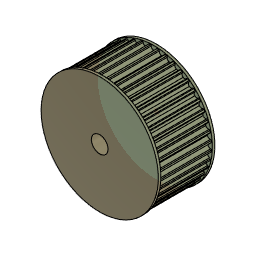
roue1 v6 (Autodesk Fusion 360 design; units mm, degrees)
Autodesk Fusion 360 part; units mm, degrees
sketch "Esquisse1" plane through (0, 0, 0) normal (0, 1, 0) x (1, 0, 0)
  circle A0 centre (0, 0) radius 35.015
  dimension "d1" = 70.03
  constraint coincident A0.centre origin
  measures "d1" diameter of A0
extrude "Extrusion1" add sketch "Esquisse1" along normal blind 1.5
sketch "Esquisse2" plane through (0, 0, 0) normal (0, 1, 0) x (1, 0, 0)
  arc A0 (-1.5243, 33.9566) -> (0, 32.385) centre (0, 33.91) ccw
  arc A1 (-29.4542, -13.4626) -> (-31.5172, -12.7295) centre (-30.8411, -14.0965) ccw
  arc A2 (-27.742, -19.6406) -> (-27.244, -17.5087) centre (-28.5269, -18.3331) ccw
  line L0 (-7.8107, 33.5477) -> (-6.8421, 33.7586)
  arc A3 (-0.0103, 32.385) -> (1.5135, 33.9571) centre (-0.0108, 33.91) ccw
  line L1 (0, 0) -> (37.4833, 0) construction
  arc A4 (-15.4926, 30.2548) -> (-16.0758, 30.4635) centre (-15.8798, 30.0921) ccw
  arc A5 (-33.9566, -1.5243) -> (-32.385, 0) centre (-33.91, 0) ccw
  line L2 (-2.9569, 34.3179) -> (-1.9681, 34.3887)
  arc A6 (-33.5477, -7.8107) -> (-33.008, -8.1146) centre (-33.1387, -7.7155) ccw
  arc A7 (33.7608, -6.8314) -> (33.396, -6.3307) centre (33.3491, -6.7481) ccw
  arc A8 (-6.3413, 33.394) -> (-6.8421, 33.7586) centre (-6.7587, 33.347) ccw
  arc A9 (-29.9883, -16.9458) -> (-29.3848, -17.0853) centre (-29.6226, -16.7392) ccw
  arc A10 (33.8279, -3.3238) -> (32.0554, -4.6089) centre (33.5648, -4.8259) ccw
  arc A11 (-13.4626, 29.4542) -> (-12.7295, 31.5172) centre (-14.0965, 30.8411) ccw
  line L3 (-33.5477, -7.8107) -> (-33.7586, -6.8421)
  arc A12 (-2.9569, 34.3179) -> (-3.3345, 33.8268) centre (-2.9208, 33.8994) ccw
  arc A13 (-32.1517, -11.0292) -> (-32.4413, -11.5768) centre (-32.0457, -11.4356) ccw
  arc A14 (-17.5173, 27.2384) -> (-17.0853, 29.3848) centre (-18.3422, 28.5211) ccw
  line L4 (-29.9883, -16.9458) -> (-30.4635, -16.0758)
  circle A15 centre (0, -33.91) radius 1.525 construction
  arc A16 (-32.385, -0.0103) -> (-33.9571, 1.5135) centre (-33.91, -0.0108) ccw
  arc A17 (33.9566, 1.5243) -> (32.385, 0) centre (33.91, 0) ccw
  arc A18 (0.0103, -32.385) -> (-1.5135, -33.9571) centre (0.0108, -33.91) ccw
  circle A19 centre (0, 0) radius 34.445 construction
  arc A20 (-30.2548, -15.4926) -> (-29.4584, -13.4532) centre (-30.8456, -14.0867) ccw
  arc A21 (3.3238, 33.8279) -> (2.946, 34.3188) centre (2.91, 33.9003) ccw
  arc A22 (9.1338, -31.0703) -> (8.1146, -33.008) centre (9.5639, -32.5334) ccw
  arc A23 (-8.1041, -33.0105) -> (-9.1239, -31.0732) centre (-9.5536, -32.5364) ccw
  arc A24 (6.3413, -33.394) -> (4.6089, -32.0554) centre (4.8259, -33.5648) ccw
  arc A25 (-24.6645, -23.3888) -> (-24.7004, -24.0072) centre (-24.3993, -23.7145) ccw
  arc A26 (31.5212, -12.7195) -> (32.0987, -12.4954) centre (31.7073, -12.343) ccw
  line L5 (34.3894, -1.9572) -> (34.3188, -2.946)
  circle A27 centre (4.8365, -33.5633) radius 1.525 construction
  arc A28 (-1.9572, -34.3894) -> (-1.5135, -33.9571) centre (-1.9333, -33.97) ccw
  arc A29 (33.8279, -3.3238) -> (34.3188, -2.946) centre (33.9003, -2.91) ccw
  arc A30 (32.4449, -11.5665) -> (32.1552, -11.019) centre (32.0493, -11.4255) ccw
  line L6 (-6.8314, -33.7608) -> (-7.8001, -33.5502)
  line L7 (-23.9994, -24.7081) -> (-24.7004, -24.0072)
  arc A31 (13.4439, 29.4627) -> (15.483, 30.2597) centre (14.0769, 30.8501) ccw
  arc A32 (15.4926, -30.2548) -> (13.4532, -29.4584) centre (14.0867, -30.8456) ccw
  line L8 (16.9458, -29.9883) -> (16.0758, -30.4635)
  arc A33 (11.5665, 32.4449) -> (11.019, 32.1552) centre (11.4255, 32.0493) ccw
  line L9 (30.4686, -16.0662) -> (29.9937, -16.9363)
  arc A34 (-17.5, -27.2496) -> (-19.6318, -27.7482) centre (-18.3241, -28.5327) ccw
  arc A35 (-26.6609, 21.0849) -> (-27.2781, 21.0324) centre (-26.9455, 20.776) ccw
  arc A36 (-27.872, 20.2388) -> (-27.7482, 19.6318) centre (-27.5322, 19.992) ccw
  arc A37 (-26.6609, 21.0849) -> (-24.4749, 21.2077) centre (-25.6275, 22.2063) ccw
  circle A38 centre (0, 0) radius 32.385 construction
  arc A39 (26.6609, -21.0849) -> (24.4749, -21.2077) centre (25.6275, -22.2063) ccw
  line L10 (27.872, -20.2388) -> (27.2781, -21.0324)
  arc A40 (26.6609, -21.0849) -> (27.2781, -21.0324) centre (26.9455, -20.776) ccw
  line L11 (0, 0) -> (5.3462, -37.1001) construction
  arc A41 (24.4817, -21.1999) -> (24.6719, -23.381) centre (25.6345, -22.1982) ccw
  arc A42 (23.3888, -24.6645) -> (21.2077, -24.4749) centre (22.2063, -25.6275) ccw
  arc A43 (-24.4817, 21.1999) -> (-24.6719, 23.381) centre (-25.6345, 22.1982) ccw
  arc A44 (19.6406, -27.742) -> (17.5087, -27.244) centre (18.3331, -28.5269) ccw
  arc A45 (19.6406, -27.742) -> (20.2476, -27.8656) centre (20.0007, -27.5258) ccw
  arc A46 (23.3888, -24.6645) -> (24.0072, -24.7004) centre (23.7145, -24.3993) ccw
  arc A47 (21.2154, -24.4682) -> (21.0933, -26.6542) centre (22.2145, -25.6204) ccw
  line L12 (0, 0) -> (0, -40) construction
  line L13 (21.0411, -27.2714) -> (20.2476, -27.8656)
  arc A48 (24.7081, -23.9994) -> (24.6719, -23.381) centre (24.4068, -23.7067) ccw
  line L14 (-27.872, 20.2388) -> (-27.2781, 21.0324)
  arc A49 (21.0411, -27.2714) -> (21.0933, -26.6542) centre (20.7845, -26.9389) ccw
  line L15 (24.7081, -23.9994) -> (24.0072, -24.7004)
  line L16 (-33.7608, 6.8314) -> (-33.5502, 7.8001)
  arc A50 (-17.076, -29.3902) -> (-16.9363, -29.9937) centre (-16.7298, -29.6279) ccw
  line L17 (-16.0662, -30.4686) -> (-16.9363, -29.9937)
  arc A51 (-3.3238, -33.8279) -> (-4.6089, -32.0554) centre (-4.8259, -33.5648) ccw
  arc A52 (16.0662, 30.4686) -> (15.483, 30.2597) centre (15.8703, 30.0971) ccw
  arc A53 (9.114, 31.0761) -> (11.019, 32.1552) centre (9.5432, 32.5394) ccw
  arc A54 (-21.1999, -24.4817) -> (-23.381, -24.6719) centre (-22.1982, -25.6345) ccw
  arc A55 (29.3902, -17.076) -> (27.244, -17.5087) centre (28.5269, -18.3331) ccw
  arc A56 (12.7195, 31.5212) -> (13.4532, 29.4584) centre (14.0867, 30.8456) ccw
  arc A57 (-21.0411, 27.2714) -> (-21.0933, 26.6542) centre (-20.7845, 26.9389) ccw
  line L18 (12.5055, -32.0947) -> (11.5768, -32.4413)
  arc A58 (-33.0105, 8.1041) -> (-33.5502, 7.8001) centre (-33.1411, 7.7049) ccw
  arc A59 (-6.8314, -33.7608) -> (-6.3307, -33.396) centre (-6.7481, -33.3491) ccw
  arc A60 (-19.6406, 27.742) -> (-17.5087, 27.244) centre (-18.3331, 28.5269) ccw
  arc A61 (-31.5212, 12.7195) -> (-29.4584, 13.4532) centre (-30.8456, 14.0867) ccw
  line L19 (11.5665, 32.4449) -> (12.4954, 32.0987)
  arc A62 (-3.3238, -33.8279) -> (-2.946, -34.3188) centre (-2.91, -33.9003) ccw
  arc A63 (6.3413, -33.394) -> (6.8421, -33.7586) centre (6.7587, -33.347) ccw
  arc A64 (-27.2496, 17.5) -> (-27.7482, 19.6318) centre (-28.5327, 18.3241) ccw
  arc A65 (-21.2154, 24.4682) -> (-21.0933, 26.6542) centre (-22.2145, 25.6204) ccw
  arc A66 (-29.4627, 13.4439) -> (-30.2597, 15.483) centre (-30.8501, 14.0769) ccw
  line L20 (6.8314, 33.7608) -> (7.8001, 33.5502)
  arc A67 (15.4926, -30.2548) -> (16.0758, -30.4635) centre (15.8798, -30.0921) ccw
  arc A68 (-34.3894, 1.9572) -> (-33.9571, 1.5135) centre (-33.97, 1.9333) ccw
  arc A69 (8.1041, 33.0105) -> (7.8001, 33.5502) centre (7.7049, 33.1411) ccw
  arc A70 (-4.5987, -32.0568) -> (-6.3307, -33.396) centre (-4.8152, -33.5664) ccw
  line L21 (-21.0411, 27.2714) -> (-20.2476, 27.8656)
  arc A71 (-33.8279, 3.3238) -> (-34.3188, 2.946) centre (-33.9003, 2.91) ccw
  arc A72 (-33.7608, 6.8314) -> (-33.396, 6.3307) centre (-33.3491, 6.7481) ccw
  arc A73 (17.076, 29.3902) -> (17.5087, 27.244) centre (18.3331, 28.5269) ccw
  line L22 (2.9569, -34.3179) -> (1.9681, -34.3887)
  line L23 (-11.5665, -32.4449) -> (-12.4954, -32.0987)
  line L24 (16.0662, 30.4686) -> (16.9363, 29.9937)
  arc A74 (-8.1041, -33.0105) -> (-7.8001, -33.5502) centre (-7.7049, -33.1411) ccw
  arc A75 (-23.3888, 24.6645) -> (-24.0072, 24.7004) centre (-23.7145, 24.3993) ccw
  arc A76 (12.5055, -32.0947) -> (12.7295, -31.5172) centre (12.3531, -31.7034) ccw
  arc A77 (4.5987, 32.0568) -> (6.3307, 33.396) centre (4.8152, 33.5664) ccw
  arc A78 (-27.2714, -21.0411) -> (-26.6542, -21.0933) centre (-26.9389, -20.7845) ccw
  arc A79 (-27.742, -19.6406) -> (-27.8656, -20.2476) centre (-27.5258, -20.0007) ccw
  arc A80 (-24.7081, 23.9994) -> (-24.6719, 23.381) centre (-24.4068, 23.7067) ccw
  line L25 (1.9572, 34.3894) -> (2.946, 34.3188)
  arc A81 (-12.7195, -31.5212) -> (-13.4532, -29.4584) centre (-14.0867, -30.8456) ccw
  arc A82 (6.8314, 33.7608) -> (6.3307, 33.396) centre (6.7481, 33.3491) ccw
  arc A83 (-17.076, -29.3902) -> (-17.5087, -27.244) centre (-18.3331, -28.5269) ccw
  line L26 (7.8107, -33.5477) -> (6.8421, -33.7586)
  arc A84 (-16.0662, -30.4686) -> (-15.483, -30.2597) centre (-15.8703, -30.0971) ccw
  arc A85 (3.3238, 33.8279) -> (4.6089, 32.0554) centre (4.8259, 33.5648) ccw
  line L27 (-27.2714, -21.0411) -> (-27.8656, -20.2476)
  arc A86 (1.5243, -33.9566) -> (1.9681, -34.3887) centre (1.9441, -33.9694) ccw
  arc A87 (17.5, 27.2496) -> (19.6318, 27.7482) centre (18.3241, 28.5327) ccw
  arc A88 (1.9572, 34.3894) -> (1.5135, 33.9571) centre (1.9333, 33.97) ccw
  arc A89 (7.8107, -33.5477) -> (8.1146, -33.008) centre (7.7155, -33.1387) ccw
  arc A90 (17.076, 29.3902) -> (16.9363, 29.9937) centre (16.7298, 29.6279) ccw
  arc A91 (4.619, -32.0539) -> (3.3345, -33.8268) centre (4.8365, -33.5633) ccw
  line L28 (-32.4449, 11.5665) -> (-32.0987, 12.4954)
  arc A92 (-19.6406, 27.742) -> (-20.2476, 27.8656) centre (-20.0007, 27.5258) ccw
  arc A93 (-13.4439, -29.4627) -> (-15.483, -30.2597) centre (-14.0769, -30.8501) ccw
  arc A94 (-32.0568, 4.5987) -> (-33.396, 6.3307) centre (-33.5664, 4.8152) ccw
  line L29 (-34.3894, 1.9572) -> (-34.3188, 2.946)
  arc A95 (1.5243, -33.9566) -> (0, -32.385) centre (0, -33.91) ccw
  circle A96 centre (1.9441, -33.9694) radius 0.42 construction
  arc A97 (8.1041, 33.0105) -> (9.1239, 31.0732) centre (9.5536, 32.5364) ccw
  arc A98 (-23.3888, 24.6645) -> (-21.2077, 24.4749) centre (-22.2063, 25.6275) ccw
  line L30 (-30.4686, 16.0662) -> (-29.9937, 16.9363)
  arc A99 (-29.3902, 17.076) -> (-29.9937, 16.9363) centre (-29.6279, 16.7298) ccw
  arc A100 (-31.0761, 9.114) -> (-32.1552, 11.019) centre (-32.5394, 9.5432) ccw
  circle A101 centre (2.9208, -33.8994) radius 0.42 construction
  arc A102 (13.4626, -29.4542) -> (12.7295, -31.5172) centre (14.0965, -30.8411) ccw
  arc A103 (-31.5212, 12.7195) -> (-32.0987, 12.4954) centre (-31.7073, 12.343) ccw
  arc A104 (2.9569, -34.3179) -> (3.3345, -33.8268) centre (2.9208, -33.8994) ccw
  arc A105 (12.7195, 31.5212) -> (12.4954, 32.0987) centre (12.343, 31.7073) ccw
  arc A106 (-21.0849, -26.6609) -> (-21.0324, -27.2781) centre (-20.776, -26.9455) ccw
  arc A107 (-33.9566, -1.5243) -> (-34.3887, -1.9681) centre (-33.9694, -1.9441) ccw
  arc A108 (-24.4682, -21.2154) -> (-26.6542, -21.0933) centre (-25.6204, -22.2145) ccw
  arc A109 (-24.6645, -23.3888) -> (-24.4749, -21.2077) centre (-25.6275, -22.2063) ccw
  arc A110 (11.0292, -32.1517) -> (11.5768, -32.4413) centre (11.4356, -32.0457) ccw
  arc A111 (-23.9994, -24.7081) -> (-23.381, -24.6719) centre (-23.7067, -24.4068) ccw
  arc A112 (32.0568, -4.5987) -> (33.396, -6.3307) centre (33.5664, -4.8152) ccw
  arc A113 (-32.0539, -4.619) -> (-33.8268, -3.3345) centre (-33.5633, -4.8365) ccw
  arc A114 (-11.0292, 32.1517) -> (-11.5768, 32.4413) centre (-11.4356, 32.0457) ccw
  arc A115 (-31.0703, -9.1338) -> (-33.008, -8.1146) centre (-32.5334, -9.5639) ccw
  arc A116 (33.0105, -8.1041) -> (31.0732, -9.1239) centre (32.5364, -9.5536) ccw
  arc A117 (27.872, -20.2388) -> (27.7482, -19.6318) centre (27.5322, -19.992) ccw
  arc A118 (-30.2548, -15.4926) -> (-30.4635, -16.0758) centre (-30.0921, -15.8798) ccw
  arc A119 (30.4686, -16.0662) -> (30.2597, -15.483) centre (30.0971, -15.8703) ccw
  line L31 (-20.2388, -27.872) -> (-21.0324, -27.2781)
  arc A120 (-9.1338, 31.0703) -> (-8.1146, 33.008) centre (-9.5639, 32.5334) ccw
  arc A121 (33.0105, -8.1041) -> (33.5502, -7.8001) centre (33.1411, -7.7049) ccw
  line L32 (32.4449, -11.5665) -> (32.0987, -12.4954)
  arc A122 (31.0761, -9.114) -> (32.1552, -11.019) centre (32.5394, -9.5432) ccw
  arc A123 (11.0292, -32.1517) -> (9.1239, -31.0732) centre (9.5536, -32.5364) ccw
  line L33 (-32.0947, -12.5055) -> (-32.4413, -11.5768)
  arc A124 (29.3902, -17.076) -> (29.9937, -16.9363) centre (29.6279, -16.7298) ccw
  arc A125 (-27.2384, -17.5173) -> (-29.3848, -17.0853) centre (-28.5211, -18.3422) ccw
  arc A126 (27.2496, -17.5) -> (27.7482, -19.6318) centre (28.5327, -18.3241) ccw
  arc A127 (-32.0947, -12.5055) -> (-31.5172, -12.7295) centre (-31.7034, -12.3531) ccw
  arc A128 (-21.0849, -26.6609) -> (-21.2077, -24.4749) centre (-22.2063, -25.6275) ccw
  arc A129 (-16.9458, 29.9883) -> (-17.0853, 29.3848) centre (-16.7392, 29.6226) ccw
  arc A130 (-20.2388, -27.872) -> (-19.6318, -27.7482) centre (-19.992, -27.5322) ccw
  line L34 (-16.9458, 29.9883) -> (-16.0758, 30.4635)
  arc A131 (-6.3413, 33.394) -> (-4.6089, 32.0554) centre (-4.8259, 33.5648) ccw
  arc A132 (-11.0292, 32.1517) -> (-9.1239, 31.0732) centre (-9.5536, 32.5364) ccw
  arc A133 (-4.619, 32.0539) -> (-3.3345, 33.8268) centre (-4.8365, 33.5633) ccw
  arc A134 (29.4627, -13.4439) -> (30.2597, -15.483) centre (30.8501, -14.0769) ccw
  arc A135 (-7.8107, 33.5477) -> (-8.1146, 33.008) centre (-7.7155, 33.1387) ccw
  arc A136 (-34.3179, -2.9569) -> (-33.8268, -3.3345) centre (-33.8994, -2.9208) ccw
  arc A137 (-12.7195, -31.5212) -> (-12.4954, -32.0987) centre (-12.343, -31.7073) ccw
  arc A138 (-33.394, -6.3413) -> (-32.0554, -4.6089) centre (-33.5648, -4.8259) ccw
  line L35 (33.7608, -6.8314) -> (33.5502, -7.8001)
  arc A139 (-32.1517, -11.0292) -> (-31.0732, -9.1239) centre (-32.5364, -9.5536) ccw
  arc A140 (31.5212, -12.7195) -> (29.4584, -13.4532) centre (30.8456, -14.0867) ccw
  arc A141 (32.385, 0.0103) -> (33.9571, -1.5135) centre (33.91, 0.0108) ccw
  arc A142 (17.5173, -27.2384) -> (17.0853, -29.3848) centre (18.3422, -28.5211) ccw
  arc A143 (-12.5055, 32.0947) -> (-12.7295, 31.5172) centre (-12.3531, 31.7034) ccw
  arc A144 (-15.4926, 30.2548) -> (-13.4532, 29.4584) centre (-14.0867, 30.8456) ccw
  arc A145 (-33.394, -6.3413) -> (-33.7586, -6.8421) centre (-33.347, -6.7587) ccw
  arc A146 (16.9458, -29.9883) -> (17.0853, -29.3848) centre (16.7392, -29.6226) ccw
  arc A147 (-11.5665, -32.4449) -> (-11.019, -32.1552) centre (-11.4255, -32.0493) ccw
  line L36 (-12.5055, 32.0947) -> (-11.5768, 32.4413)
  line L37 (-1.9572, -34.3894) -> (-2.946, -34.3188)
  line L38 (-34.3179, -2.9569) -> (-34.3887, -1.9681)
  arc A148 (34.3894, -1.9572) -> (33.9571, -1.5135) centre (33.97, -1.9333) ccw
  arc A149 (-1.5243, 33.9566) -> (-1.9681, 34.3887) centre (-1.9441, 33.9694) ccw
  arc A150 (-9.114, -31.0761) -> (-11.019, -32.1552) centre (-9.5432, -32.5394) ccw
  arc A151 (31.0703, 9.1338) -> (33.008, 8.1146) centre (32.5334, 9.5639) ccw
  arc A152 (32.0539, 4.619) -> (33.8268, 3.3345) centre (33.5633, 4.8365) ccw
  arc A153 (24.6645, 23.3888) -> (24.4749, 21.2077) centre (25.6275, 22.2063) ccw
  arc A154 (21.1999, 24.4817) -> (23.381, 24.6719) centre (22.1982, 25.6345) ccw
  line L39 (20.2388, 27.872) -> (21.0324, 27.2781)
  arc A155 (33.394, 6.3413) -> (33.7586, 6.8421) centre (33.347, 6.7587) ccw
  arc A156 (29.9883, 16.9458) -> (29.3848, 17.0853) centre (29.6226, 16.7392) ccw
  arc A157 (21.0849, 26.6609) -> (21.0324, 27.2781) centre (20.776, 26.9455) ccw
  arc A158 (33.5477, 7.8107) -> (33.008, 8.1146) centre (33.1387, 7.7155) ccw
  arc A159 (33.9566, 1.5243) -> (34.3887, 1.9681) centre (33.9694, 1.9441) ccw
  arc A160 (-33.0105, 8.1041) -> (-31.0732, 9.1239) centre (-32.5364, 9.5536) ccw
  arc A161 (-32.4449, 11.5665) -> (-32.1552, 11.019) centre (-32.0493, 11.4255) ccw
  arc A162 (-33.8279, 3.3238) -> (-32.0554, 4.6089) centre (-33.5648, 4.8259) ccw
  arc A163 (29.4542, 13.4626) -> (31.5172, 12.7295) centre (30.8411, 14.0965) ccw
  arc A164 (-29.3902, 17.076) -> (-27.244, 17.5087) centre (-28.5269, 18.3331) ccw
  line L40 (34.3179, 2.9569) -> (34.3887, 1.9681)
  line L41 (-24.7081, 23.9994) -> (-24.0072, 24.7004)
  arc A165 (27.742, 19.6406) -> (27.244, 17.5087) centre (28.5269, 18.3331) ccw
  arc A166 (33.394, 6.3413) -> (32.0554, 4.6089) centre (33.5648, 4.8259) ccw
  arc A167 (20.2388, 27.872) -> (19.6318, 27.7482) centre (19.992, 27.5322) ccw
  arc A168 (23.9994, 24.7081) -> (23.381, 24.6719) centre (23.7067, 24.4068) ccw
  arc A169 (21.0849, 26.6609) -> (21.2077, 24.4749) centre (22.2063, 25.6275) ccw
  arc A170 (-30.4686, 16.0662) -> (-30.2597, 15.483) centre (-30.0971, 15.8703) ccw
  line L42 (23.9994, 24.7081) -> (24.7004, 24.0072)
  line L43 (27.2714, 21.0411) -> (27.8656, 20.2476)
  arc A171 (27.742, 19.6406) -> (27.8656, 20.2476) centre (27.5258, 20.0007) ccw
  arc A172 (32.0947, 12.5055) -> (31.5172, 12.7295) centre (31.7034, 12.3531) ccw
  arc A173 (32.1517, 11.0292) -> (32.4413, 11.5768) centre (32.0457, 11.4356) ccw
  arc A174 (24.4682, 21.2154) -> (26.6542, 21.0933) centre (25.6204, 22.2145) ccw
  arc A175 (34.3179, 2.9569) -> (33.8268, 3.3345) centre (33.8994, 2.9208) ccw
  line L44 (33.5477, 7.8107) -> (33.7586, 6.8421)
  line L45 (32.0947, 12.5055) -> (32.4413, 11.5768)
  arc A176 (30.2548, 15.4926) -> (29.4584, 13.4532) centre (30.8456, 14.0867) ccw
  line L46 (29.9883, 16.9458) -> (30.4635, 16.0758)
  arc A177 (27.2714, 21.0411) -> (26.6542, 21.0933) centre (26.9389, 20.7845) ccw
  arc A178 (24.6645, 23.3888) -> (24.7004, 24.0072) centre (24.3993, 23.7145) ccw
  arc A179 (27.2384, 17.5173) -> (29.3848, 17.0853) centre (28.5211, 18.3422) ccw
  arc A180 (30.2548, 15.4926) -> (30.4635, 16.0758) centre (30.0921, 15.8798) ccw
  arc A181 (32.1517, 11.0292) -> (31.0732, 9.1239) centre (32.5364, 9.5536) ccw
  dimension "d5" = 360
  dimension "d6" = 68.89
  dimension "d7" = 64.77
  dimension "d8" = 3.05
  dimension "d9" = 0.84
  dimension "d10" = 81.8
  dimension "d11" = 3.05
  dimension "d12" = 0.84
  constraint coincident L1.start A19.centre
  constraint concentric A19 A38
  constraint vertical L12
  constraint tangent A19 A96
  constraint tangent A15 A96
  constraint horizontal L1
  constraint tangent A27 A101
  constraint tangent A19 A101
  constraint coincident A86.start A96
  constraint coincident A95.end A38
  constraint coincident A95.end L12
  constraint coincident L22.end A19
  constraint coincident A86.centre A96.centre
  constraint coincident A91.end A27
  constraint coincident L22.start A101
  constraint coincident A101.centre A104.centre
  constraint coincident A91.start L11
  constraint coincident A27.centre A91.centre
  measures "d6" diameter of A19
  measures "d7" diameter of A38
  measures "d8" diameter of A15
  measures "d9" diameter of A96
  measures "d10" angle of L1 L11
  measures "d11" diameter of A27
  measures "d12" diameter of A101
extrude "Extrusion2" add sketch "Esquisse2" against normal blind 30.8
sketch "Esquisse3" plane through (0, -30.8, 0) normal (0, -1, 0) x (1, 0, 0)
  arc A0 (31.5172, -12.7295) -> (32.0947, -12.5055) centre (31.7034, -12.3531) ccw
  line L0 (32.0947, -12.5055) -> (32.4413, -11.5768)
  arc A1 (32.4413, -11.5768) -> (32.1517, -11.0292) centre (32.0457, -11.4356) ccw
  arc A2 (31.0717, -9.1288) -> (32.1517, -11.0292) centre (32.5364, -9.5536) ccw
  arc A3 (33.008, -8.1146) -> (31.0717, -9.1288) centre (32.5334, -9.5639) ccw
  arc A4 (33.008, -8.1146) -> (33.5477, -7.8107) centre (33.1387, -7.7155) ccw
  line L1 (33.5477, -7.8107) -> (33.7586, -6.8421)
  arc A5 (33.7586, -6.8421) -> (33.394, -6.3413) centre (33.347, -6.7587) ccw
  arc A6 (32.0546, -4.614) -> (33.394, -6.3413) centre (33.5648, -4.8259) ccw
  arc A7 (33.8268, -3.3345) -> (32.0546, -4.614) centre (33.5633, -4.8365) ccw
  arc A8 (33.8268, -3.3345) -> (34.3179, -2.9569) centre (33.8994, -2.9208) ccw
  line L2 (34.3179, -2.9569) -> (34.3887, -1.9681)
  arc A9 (34.3887, -1.9681) -> (33.9566, -1.5243) centre (33.9694, -1.9441) ccw
  arc A10 (32.385, -0.0051) -> (33.9566, -1.5243) centre (33.91, 0) ccw
  arc A11 (33.9571, 1.5135) -> (32.385, -0.0051) centre (33.91, -0.0108) ccw
  arc A12 (33.9571, 1.5135) -> (34.3894, 1.9572) centre (33.97, 1.9333) ccw
  line L3 (34.3894, 1.9572) -> (34.3188, 2.946)
  arc A13 (34.3188, 2.946) -> (33.8279, 3.3238) centre (33.9003, 2.91) ccw
  arc A14 (32.0561, 4.6038) -> (33.8279, 3.3238) centre (33.5648, 4.8259) ccw
  arc A15 (33.396, 6.3307) -> (32.0561, 4.6038) centre (33.5664, 4.8152) ccw
  arc A16 (33.396, 6.3307) -> (33.7608, 6.8314) centre (33.3491, 6.7481) ccw
  line L4 (33.7608, 6.8314) -> (33.5502, 7.8001)
  arc A17 (33.5502, 7.8001) -> (33.0105, 8.1041) centre (33.1411, 7.7049) ccw
  arc A18 (31.0746, 9.119) -> (33.0105, 8.1041) centre (32.5364, 9.5536) ccw
  arc A19 (32.1552, 11.019) -> (31.0746, 9.119) centre (32.5394, 9.5432) ccw
  arc A20 (32.1552, 11.019) -> (32.4449, 11.5665) centre (32.0493, 11.4255) ccw
  line L5 (32.4449, 11.5665) -> (32.0987, 12.4954)
  arc A21 (32.0987, 12.4954) -> (31.5212, 12.7195) centre (31.7073, 12.343) ccw
  arc A22 (29.4606, 13.4485) -> (31.5212, 12.7195) centre (30.8456, 14.0867) ccw
  arc A23 (30.2597, 15.483) -> (29.4606, 13.4485) centre (30.8501, 14.0769) ccw
  arc A24 (30.2597, 15.483) -> (30.4686, 16.0662) centre (30.0971, 15.8703) ccw
  line L6 (30.4686, 16.0662) -> (29.9937, 16.9363)
  arc A25 (29.9937, 16.9363) -> (29.3902, 17.076) centre (29.6279, 16.7298) ccw
  arc A26 (27.2468, 17.5043) -> (29.3902, 17.076) centre (28.5269, 18.3331) ccw
  arc A27 (27.7482, 19.6318) -> (27.2468, 17.5043) centre (28.5327, 18.3241) ccw
  arc A28 (27.7482, 19.6318) -> (27.872, 20.2388) centre (27.5322, 19.992) ccw
  line L7 (27.872, 20.2388) -> (27.2781, 21.0324)
  arc A29 (27.2781, 21.0324) -> (26.6609, 21.0849) centre (26.9455, 20.776) ccw
  arc A30 (24.4783, 21.2038) -> (26.6609, 21.0849) centre (25.6275, 22.2063) ccw
  arc A31 (24.6719, 23.381) -> (24.4783, 21.2038) centre (25.6345, 22.1982) ccw
  arc A32 (24.6719, 23.381) -> (24.7081, 23.9994) centre (24.4068, 23.7067) ccw
  line L8 (24.7081, 23.9994) -> (24.0072, 24.7004)
  arc A33 (24.0072, 24.7004) -> (23.3888, 24.6645) centre (23.7145, 24.3993) ccw
  arc A34 (21.2116, 24.4716) -> (23.3888, 24.6645) centre (22.2063, 25.6275) ccw
  arc A35 (21.0933, 26.6542) -> (21.2116, 24.4716) centre (22.2145, 25.6204) ccw
  arc A36 (21.0933, 26.6542) -> (21.0411, 27.2714) centre (20.7845, 26.9389) ccw
  line L9 (21.0411, 27.2714) -> (20.2476, 27.8656)
  arc A37 (20.2476, 27.8656) -> (19.6406, 27.742) centre (20.0007, 27.5258) ccw
  arc A38 (17.513, 27.2412) -> (19.6406, 27.742) centre (18.3331, 28.5269) ccw
  arc A39 (17.0853, 29.3848) -> (17.513, 27.2412) centre (18.3422, 28.5211) ccw
  arc A40 (17.0853, 29.3848) -> (16.9458, 29.9883) centre (16.7392, 29.6226) ccw
  line L10 (16.9458, 29.9883) -> (16.0758, 30.4635)
  arc A41 (16.0758, 30.4635) -> (15.4926, 30.2548) centre (15.8798, 30.0921) ccw
  arc A42 (13.4579, 29.4563) -> (15.4926, 30.2548) centre (14.0867, 30.8456) ccw
  arc A43 (12.7295, 31.5172) -> (13.4579, 29.4563) centre (14.0965, 30.8411) ccw
  arc A44 (12.7295, 31.5172) -> (12.5055, 32.0947) centre (12.3531, 31.7034) ccw
  line L11 (12.5055, 32.0947) -> (11.5768, 32.4413)
  arc A45 (11.5768, 32.4413) -> (11.0292, 32.1517) centre (11.4356, 32.0457) ccw
  arc A46 (9.1288, 31.0717) -> (11.0292, 32.1517) centre (9.5536, 32.5364) ccw
  arc A47 (8.1146, 33.008) -> (9.1288, 31.0717) centre (9.5639, 32.5334) ccw
  arc A48 (8.1146, 33.008) -> (7.8107, 33.5477) centre (7.7155, 33.1387) ccw
  line L12 (7.8107, 33.5477) -> (6.8421, 33.7586)
  arc A49 (6.8421, 33.7586) -> (6.3413, 33.394) centre (6.7587, 33.347) ccw
  arc A50 (4.614, 32.0546) -> (6.3413, 33.394) centre (4.8259, 33.5648) ccw
  arc A51 (3.3345, 33.8268) -> (4.614, 32.0546) centre (4.8365, 33.5633) ccw
  arc A52 (3.3345, 33.8268) -> (2.9569, 34.3179) centre (2.9208, 33.8994) ccw
  line L13 (2.9569, 34.3179) -> (1.9681, 34.3887)
  arc A53 (1.9681, 34.3887) -> (1.5243, 33.9566) centre (1.9441, 33.9694) ccw
  arc A54 (0.0051, 32.385) -> (1.5243, 33.9566) centre (0, 33.91) ccw
  arc A55 (-1.5135, 33.9571) -> (0.0051, 32.385) centre (0.0108, 33.91) ccw
  arc A56 (-1.5135, 33.9571) -> (-1.9572, 34.3894) centre (-1.9333, 33.97) ccw
  line L14 (-1.9572, 34.3894) -> (-2.946, 34.3188)
  arc A57 (-2.946, 34.3188) -> (-3.3238, 33.8279) centre (-2.91, 33.9003) ccw
  arc A58 (-4.6038, 32.0561) -> (-3.3238, 33.8279) centre (-4.8259, 33.5648) ccw
  arc A59 (-6.3307, 33.396) -> (-4.6038, 32.0561) centre (-4.8152, 33.5664) ccw
  arc A60 (-6.3307, 33.396) -> (-6.8314, 33.7608) centre (-6.7481, 33.3491) ccw
  line L15 (-6.8314, 33.7608) -> (-7.8001, 33.5502)
  arc A61 (-7.8001, 33.5502) -> (-8.1041, 33.0105) centre (-7.7049, 33.1411) ccw
  arc A62 (-9.119, 31.0746) -> (-8.1041, 33.0105) centre (-9.5536, 32.5364) ccw
  arc A63 (-11.019, 32.1552) -> (-9.119, 31.0746) centre (-9.5432, 32.5394) ccw
  arc A64 (-11.019, 32.1552) -> (-11.5665, 32.4449) centre (-11.4255, 32.0493) ccw
  line L16 (-11.5665, 32.4449) -> (-12.4954, 32.0987)
  arc A65 (-12.4954, 32.0987) -> (-12.7195, 31.5212) centre (-12.343, 31.7073) ccw
  arc A66 (-13.4485, 29.4606) -> (-12.7195, 31.5212) centre (-14.0867, 30.8456) ccw
  arc A67 (-15.483, 30.2597) -> (-13.4485, 29.4606) centre (-14.0769, 30.8501) ccw
  arc A68 (-15.483, 30.2597) -> (-16.0662, 30.4686) centre (-15.8703, 30.0971) ccw
  line L17 (-16.0662, 30.4686) -> (-16.9363, 29.9937)
  arc A69 (-16.9363, 29.9937) -> (-17.076, 29.3902) centre (-16.7298, 29.6279) ccw
  arc A70 (-17.5043, 27.2468) -> (-17.076, 29.3902) centre (-18.3331, 28.5269) ccw
  arc A71 (-19.6318, 27.7482) -> (-17.5043, 27.2468) centre (-18.3241, 28.5327) ccw
  arc A72 (-19.6318, 27.7482) -> (-20.2388, 27.872) centre (-19.992, 27.5322) ccw
  line L18 (-20.2388, 27.872) -> (-21.0324, 27.2781)
  arc A73 (-21.0324, 27.2781) -> (-21.0849, 26.6609) centre (-20.776, 26.9455) ccw
  arc A74 (-21.2038, 24.4783) -> (-21.0849, 26.6609) centre (-22.2063, 25.6275) ccw
  arc A75 (-23.381, 24.6719) -> (-21.2038, 24.4783) centre (-22.1982, 25.6345) ccw
  arc A76 (-23.381, 24.6719) -> (-23.9994, 24.7081) centre (-23.7067, 24.4068) ccw
  line L19 (-23.9994, 24.7081) -> (-24.7004, 24.0072)
  arc A77 (-24.7004, 24.0072) -> (-24.6645, 23.3888) centre (-24.3993, 23.7145) ccw
  arc A78 (-24.4716, 21.2116) -> (-24.6645, 23.3888) centre (-25.6275, 22.2063) ccw
  arc A79 (-26.6542, 21.0933) -> (-24.4716, 21.2116) centre (-25.6204, 22.2145) ccw
  arc A80 (-26.6542, 21.0933) -> (-27.2714, 21.0411) centre (-26.9389, 20.7845) ccw
  line L20 (-27.2714, 21.0411) -> (-27.8656, 20.2476)
  arc A81 (-27.8656, 20.2476) -> (-27.742, 19.6406) centre (-27.5258, 20.0007) ccw
  arc A82 (-27.2412, 17.513) -> (-27.742, 19.6406) centre (-28.5269, 18.3331) ccw
  arc A83 (-29.3848, 17.0853) -> (-27.2412, 17.513) centre (-28.5211, 18.3422) ccw
  arc A84 (-29.3848, 17.0853) -> (-29.9883, 16.9458) centre (-29.6226, 16.7392) ccw
  line L21 (-29.9883, 16.9458) -> (-30.4635, 16.0758)
  arc A85 (-30.4635, 16.0758) -> (-30.2548, 15.4926) centre (-30.0921, 15.8798) ccw
  arc A86 (-29.4563, 13.4579) -> (-30.2548, 15.4926) centre (-30.8456, 14.0867) ccw
  arc A87 (-31.5172, 12.7295) -> (-29.4563, 13.4579) centre (-30.8411, 14.0965) ccw
  arc A88 (-31.5172, 12.7295) -> (-32.0947, 12.5055) centre (-31.7034, 12.3531) ccw
  line L22 (-32.0947, 12.5055) -> (-32.4413, 11.5768)
  arc A89 (-32.4413, 11.5768) -> (-32.1517, 11.0292) centre (-32.0457, 11.4356) ccw
  arc A90 (-31.0717, 9.1288) -> (-32.1517, 11.0292) centre (-32.5364, 9.5536) ccw
  arc A91 (-33.008, 8.1146) -> (-31.0717, 9.1288) centre (-32.5334, 9.5639) ccw
  arc A92 (-33.008, 8.1146) -> (-33.5477, 7.8107) centre (-33.1387, 7.7155) ccw
  line L23 (-33.5477, 7.8107) -> (-33.7586, 6.8421)
  arc A93 (-33.7586, 6.8421) -> (-33.394, 6.3413) centre (-33.347, 6.7587) ccw
  arc A94 (-32.0546, 4.614) -> (-33.394, 6.3413) centre (-33.5648, 4.8259) ccw
  arc A95 (-33.8268, 3.3345) -> (-32.0546, 4.614) centre (-33.5633, 4.8365) ccw
  arc A96 (-33.8268, 3.3345) -> (-34.3179, 2.9569) centre (-33.8994, 2.9208) ccw
  line L24 (-34.3179, 2.9569) -> (-34.3887, 1.9681)
  arc A97 (-34.3887, 1.9681) -> (-33.9566, 1.5243) centre (-33.9694, 1.9441) ccw
  arc A98 (-32.385, 0.0051) -> (-33.9566, 1.5243) centre (-33.91, 0) ccw
  arc A99 (-33.9571, -1.5135) -> (-32.385, 0.0051) centre (-33.91, 0.0108) ccw
  arc A100 (-33.9571, -1.5135) -> (-34.3894, -1.9572) centre (-33.97, -1.9333) ccw
  line L25 (-34.3894, -1.9572) -> (-34.3188, -2.946)
  arc A101 (-34.3188, -2.946) -> (-33.8279, -3.3238) centre (-33.9003, -2.91) ccw
  arc A102 (-32.0561, -4.6038) -> (-33.8279, -3.3238) centre (-33.5648, -4.8259) ccw
  arc A103 (-33.396, -6.3307) -> (-32.0561, -4.6038) centre (-33.5664, -4.8152) ccw
  arc A104 (-33.396, -6.3307) -> (-33.7608, -6.8314) centre (-33.3491, -6.7481) ccw
  line L26 (-33.7608, -6.8314) -> (-33.5502, -7.8001)
  arc A105 (-33.5502, -7.8001) -> (-33.0105, -8.1041) centre (-33.1411, -7.7049) ccw
  arc A106 (-31.0746, -9.119) -> (-33.0105, -8.1041) centre (-32.5364, -9.5536) ccw
  arc A107 (-32.1552, -11.019) -> (-31.0746, -9.119) centre (-32.5394, -9.5432) ccw
  arc A108 (-32.1552, -11.019) -> (-32.4449, -11.5665) centre (-32.0493, -11.4255) ccw
  line L27 (-32.4449, -11.5665) -> (-32.0987, -12.4954)
  arc A109 (-32.0987, -12.4954) -> (-31.5212, -12.7195) centre (-31.7073, -12.343) ccw
  arc A110 (-29.4606, -13.4485) -> (-31.5212, -12.7195) centre (-30.8456, -14.0867) ccw
  arc A111 (-30.2597, -15.483) -> (-29.4606, -13.4485) centre (-30.8501, -14.0769) ccw
  arc A112 (-30.2597, -15.483) -> (-30.4686, -16.0662) centre (-30.0971, -15.8703) ccw
  line L28 (-30.4686, -16.0662) -> (-29.9937, -16.9363)
  arc A113 (-29.9937, -16.9363) -> (-29.3902, -17.076) centre (-29.6279, -16.7298) ccw
  arc A114 (-27.2468, -17.5043) -> (-29.3902, -17.076) centre (-28.5269, -18.3331) ccw
  arc A115 (-27.7482, -19.6318) -> (-27.2468, -17.5043) centre (-28.5327, -18.3241) ccw
  arc A116 (-27.7482, -19.6318) -> (-27.872, -20.2388) centre (-27.5322, -19.992) ccw
  line L29 (-27.872, -20.2388) -> (-27.2781, -21.0324)
  arc A117 (-27.2781, -21.0324) -> (-26.6609, -21.0849) centre (-26.9455, -20.776) ccw
  arc A118 (-24.4783, -21.2038) -> (-26.6609, -21.0849) centre (-25.6275, -22.2063) ccw
  arc A119 (-24.6719, -23.381) -> (-24.4783, -21.2038) centre (-25.6345, -22.1982) ccw
  arc A120 (-24.6719, -23.381) -> (-24.7081, -23.9994) centre (-24.4068, -23.7067) ccw
  line L30 (-24.7081, -23.9994) -> (-24.0072, -24.7004)
  arc A121 (-24.0072, -24.7004) -> (-23.3888, -24.6645) centre (-23.7145, -24.3993) ccw
  arc A122 (-21.2116, -24.4716) -> (-23.3888, -24.6645) centre (-22.2063, -25.6275) ccw
  arc A123 (-21.0933, -26.6542) -> (-21.2116, -24.4716) centre (-22.2145, -25.6204) ccw
  arc A124 (-21.0933, -26.6542) -> (-21.0411, -27.2714) centre (-20.7845, -26.9389) ccw
  line L31 (-21.0411, -27.2714) -> (-20.2476, -27.8656)
  arc A125 (-20.2476, -27.8656) -> (-19.6406, -27.742) centre (-20.0007, -27.5258) ccw
  arc A126 (-17.513, -27.2412) -> (-19.6406, -27.742) centre (-18.3331, -28.5269) ccw
  arc A127 (-17.0853, -29.3848) -> (-17.513, -27.2412) centre (-18.3422, -28.5211) ccw
  arc A128 (-17.0853, -29.3848) -> (-16.9458, -29.9883) centre (-16.7392, -29.6226) ccw
  line L32 (-16.9458, -29.9883) -> (-16.0758, -30.4635)
  arc A129 (-16.0758, -30.4635) -> (-15.4926, -30.2548) centre (-15.8798, -30.0921) ccw
  arc A130 (-13.4579, -29.4563) -> (-15.4926, -30.2548) centre (-14.0867, -30.8456) ccw
  arc A131 (-12.7295, -31.5172) -> (-13.4579, -29.4563) centre (-14.0965, -30.8411) ccw
  arc A132 (-12.7295, -31.5172) -> (-12.5055, -32.0947) centre (-12.3531, -31.7034) ccw
  line L33 (-12.5055, -32.0947) -> (-11.5768, -32.4413)
  arc A133 (-11.5768, -32.4413) -> (-11.0292, -32.1517) centre (-11.4356, -32.0457) ccw
  arc A134 (-9.1288, -31.0717) -> (-11.0292, -32.1517) centre (-9.5536, -32.5364) ccw
  arc A135 (-8.1146, -33.008) -> (-9.1288, -31.0717) centre (-9.5639, -32.5334) ccw
  arc A136 (-8.1146, -33.008) -> (-7.8107, -33.5477) centre (-7.7155, -33.1387) ccw
  line L34 (-7.8107, -33.5477) -> (-6.8421, -33.7586)
  arc A137 (-6.8421, -33.7586) -> (-6.3413, -33.394) centre (-6.7587, -33.347) ccw
  arc A138 (-4.614, -32.0546) -> (-6.3413, -33.394) centre (-4.8259, -33.5648) ccw
  arc A139 (-3.3345, -33.8268) -> (-4.614, -32.0546) centre (-4.8365, -33.5633) ccw
  arc A140 (-3.3345, -33.8268) -> (-2.9569, -34.3179) centre (-2.9208, -33.8994) ccw
  line L35 (-2.9569, -34.3179) -> (-1.9681, -34.3887)
  arc A141 (-1.9681, -34.3887) -> (-1.5243, -33.9566) centre (-1.9441, -33.9694) ccw
  arc A142 (-0.0051, -32.385) -> (-1.5243, -33.9566) centre (0, -33.91) ccw
  arc A143 (1.5135, -33.9571) -> (-0.0051, -32.385) centre (-0.0108, -33.91) ccw
  arc A144 (1.5135, -33.9571) -> (1.9572, -34.3894) centre (1.9333, -33.97) ccw
  line L36 (1.9572, -34.3894) -> (2.946, -34.3188)
  arc A145 (2.946, -34.3188) -> (3.3238, -33.8279) centre (2.91, -33.9003) ccw
  arc A146 (4.6038, -32.0561) -> (3.3238, -33.8279) centre (4.8259, -33.5648) ccw
  arc A147 (6.3307, -33.396) -> (4.6038, -32.0561) centre (4.8152, -33.5664) ccw
  arc A148 (6.3307, -33.396) -> (6.8314, -33.7608) centre (6.7481, -33.3491) ccw
  line L37 (6.8314, -33.7608) -> (7.8001, -33.5502)
  arc A149 (7.8001, -33.5502) -> (8.1041, -33.0105) centre (7.7049, -33.1411) ccw
  arc A150 (9.119, -31.0746) -> (8.1041, -33.0105) centre (9.5536, -32.5364) ccw
  arc A151 (11.019, -32.1552) -> (9.119, -31.0746) centre (9.5432, -32.5394) ccw
  arc A152 (11.019, -32.1552) -> (11.5665, -32.4449) centre (11.4255, -32.0493) ccw
  line L38 (11.5665, -32.4449) -> (12.4954, -32.0987)
  arc A153 (12.4954, -32.0987) -> (12.7195, -31.5212) centre (12.343, -31.7073) ccw
  arc A154 (13.4485, -29.4606) -> (12.7195, -31.5212) centre (14.0867, -30.8456) ccw
  arc A155 (15.483, -30.2597) -> (13.4485, -29.4606) centre (14.0769, -30.8501) ccw
  arc A156 (15.483, -30.2597) -> (16.0662, -30.4686) centre (15.8703, -30.0971) ccw
  line L39 (16.0662, -30.4686) -> (16.9363, -29.9937)
  arc A157 (16.9363, -29.9937) -> (17.076, -29.3902) centre (16.7298, -29.6279) ccw
  arc A158 (17.5043, -27.2468) -> (17.076, -29.3902) centre (18.3331, -28.5269) ccw
  arc A159 (19.6318, -27.7482) -> (17.5043, -27.2468) centre (18.3241, -28.5327) ccw
  arc A160 (19.6318, -27.7482) -> (20.2388, -27.872) centre (19.992, -27.5322) ccw
  line L40 (20.2388, -27.872) -> (21.0324, -27.2781)
  arc A161 (21.0324, -27.2781) -> (21.0849, -26.6609) centre (20.776, -26.9455) ccw
  arc A162 (21.2038, -24.4783) -> (21.0849, -26.6609) centre (22.2063, -25.6275) ccw
  arc A163 (23.381, -24.6719) -> (21.2038, -24.4783) centre (22.1982, -25.6345) ccw
  arc A164 (23.381, -24.6719) -> (23.9994, -24.7081) centre (23.7067, -24.4068) ccw
  line L41 (23.9994, -24.7081) -> (24.7004, -24.0072)
  arc A165 (24.7004, -24.0072) -> (24.6645, -23.3888) centre (24.3993, -23.7145) ccw
  arc A166 (24.4716, -21.2116) -> (24.6645, -23.3888) centre (25.6275, -22.2063) ccw
  arc A167 (26.6542, -21.0933) -> (24.4716, -21.2116) centre (25.6204, -22.2145) ccw
  arc A168 (26.6542, -21.0933) -> (27.2714, -21.0411) centre (26.9389, -20.7845) ccw
  line L42 (27.2714, -21.0411) -> (27.8656, -20.2476)
  arc A169 (27.8656, -20.2476) -> (27.742, -19.6406) centre (27.5258, -20.0007) ccw
  arc A170 (27.2412, -17.513) -> (27.742, -19.6406) centre (28.5269, -18.3331) ccw
  arc A171 (29.3848, -17.0853) -> (27.2412, -17.513) centre (28.5211, -18.3422) ccw
  arc A172 (29.3848, -17.0853) -> (29.9883, -16.9458) centre (29.6226, -16.7392) ccw
  line L43 (29.9883, -16.9458) -> (30.4635, -16.0758)
  arc A173 (30.4635, -16.0758) -> (30.2548, -15.4926) centre (30.0921, -15.8798) ccw
  arc A174 (29.4563, -13.4579) -> (30.2548, -15.4926) centre (30.8456, -14.0867) ccw
  arc A175 (31.5172, -12.7295) -> (29.4563, -13.4579) centre (30.8411, -14.0965) ccw
  circle A176 centre (0, 0) radius 35.015
  dimension "d15" = 70.03
  constraint coincident A176.centre origin
  measures "d15" diameter of A176
extrude "Extrusion3" add sketch "Esquisse3" 1 faces at (-11.3558, -30.8, -4.5943) along normal blind 1.5 contours A0 L0 A1 A2 A3 A4 L1 A5 A6 A7 A8 L2 A9 A10 A11 A12 L3 A13 A14 A15 A16 L4 A17 A18 A19 A20 L5 A21 A22 A23 A24 L6 A25 A26 A27 A28 L7 A29 A30 A31 A32 L8 A33 A34 A35 A36 L9 A37 A38 A39 A40 L10 A41 A42 A43 A44 L11 A45 A46 A47 A48 L12 A49 A50 A51 A52 L13 A53 A54 A55 A56 L14 A57 A58 A59 A60 L15 A61 A62 A63 A64 L16 A65 A66 A67 A68 L17 A69 A70 A71 A72 L18 A73 A74 A75 A76 L19 A77 A78 A79 A80 L20 A81 A82 A83 A84 L21 A85 A86 A87 A88 L22 A89 A90 A91 A92 L23 A93 A94 A95 A96 L24 A97 A98 A99 A100 L25 A101 A102 A103 A104 L26 A105 A106 A107 A108 L27 A109 A110 A111 A112 L28 A113 A114 A115 A116 L29 A117 A118 A119 A120 L30 A121 A122 A123 A124 L31 A125 A126 A127 A128 L32 A129 A130 A131 A132 L33 A133 A134 A135 A136 L34 A137 A138 A139 A140 L35 A141 A142 A143 A144 L36 A145 A146 A147 A148 L37 A149 A150 A151 A152 L38 A153 A154 A155 A156 L39 A157 A158 A159 A160 L40 A161 A162 A163 A164 L41 A165 A166 A167 A168 L42 A169 A170 A171 A172 L43 A173 A174 A175 | A176
sketch "Esquisse4" plane through (0, 1.5, 0) normal (0, 1, 0) x (-1, 0, 0)
  circle A0 centre (0, 0) radius 35.015
  circle A1 centre (0, 0) radius 1.6
  dimension "d18" = 3.2
  constraint concentric A0 A1
  measures "d18" diameter of A1
extrude "Extrusion4" cut sketch "Esquisse4" against normal blind 9 contours A1
sketch "Esquisse5" plane through (0, -32.3, 0) normal (0, -1, 0) x (1, 0, 0)
  circle A0 centre (0, 0) radius 35.015
  circle A1 centre (0, 0) radius 5
  dimension "d21" = 10
  constraint concentric A0 A1
  measures "d21" diameter of A1
extrude "Extrusion5" cut sketch "Esquisse5" against normal blind 24 contours A1
